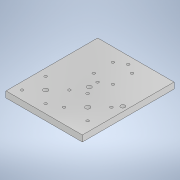
# Autodesk Inventor part: 14_XY_Plate
Saved by Autodesk Inventor 2022.2 (Build 262287010, 287A)
## iProperties
Created: 2022-04-30
Part Number: 14_XY_Plate
Material: Aluminium 6061
Document SubType Name: Modeling
Designer: MXBD
Density: 2.7 g/cm^3
Appearance: Aluminium - dunkel
Author: MXBD
Autodesk Inventor part; units mm, degrees
ref_plane "YZ Plane" through (0, 0, 0) normal (1, 0, 0) x (0, 1, 0)
ref_plane "XZ Plane" through (0, 0, 0) normal (0, 1, 0) x (-1, 0, 0)
ref_plane "XY Plane" through (0, 0, 0) normal (0, 0, 1) x (1, 0, 0)
sketch "Skizze1" plane through (0, 0, 0) normal (0, 1, 0) x (-1, 0, 0)
  line L0 (50, -60) -> (-50, -60)
  line L1 (-50, -60) -> (-50, 60)
  line L2 (-50, 60) -> (50, 60)
  line L3 (50, 60) -> (50, -60)
  line L4 (50, -60) -> (-50, 60) construction
  line L5 (-50, -60) -> (50, 60) construction
  point P0 (0, 0)
  dimension "d0" = 100
  dimension "d1" = 120
  constraints: 12 end point, 2 midpoint, 2 parallel, 1 horizontal, 1 perpendicular
  measures "d0" distance of L1.end L2.end
  measures "d1" distance of L0.end L1.end
extrude "Extrusion1" add sketch "Skizze1" along normal blind 8
sketch "Skizze2" plane through (0, 8, 0) normal (0, 1, 0) x (1, 0, 0)
  line L0 (-50, -60) -> (50, -60) projected
  line L1 (0, -60) -> (0, 152.9688)
  line L2 (50, 60) -> (-50, 60) projected
  point P0 (0, 0)
  point P1 (0, 10)
  point P2 (0, 50)
  dimension "d4" = 40
  dimension "d5" = 10
  constraints: 2 end point, 2 point on line, 1 midpoint, 1 vertical
  measures "d4" distance of point (0, 50) point (0, 10)
  measures "d5" distance from line of L2 point (0, 50)
hole "Rail_through_holes" at (0, 8, -10) at (0, 8, -50) direction (0, -1, 0) diameter 3.4 end through all clearance for "Inbusschraube ISO 4762" size "M3" standard "ISO"
sketch "Skizze3" plane through (0, 8, 0) normal (0, 1, 0) x (1, 0, 0)
  line L0 (-50, -60) -> (50, -60) projected
  line L1 (0, -60) -> (0, 60)
  line L2 (50, 60) -> (-50, 60) projected
  line L3 (12.5, 17.5) -> (-12.5, 17.5) construction
  line L4 (-12.5, 17.5) -> (-12.5, 42.5) construction
  line L5 (-12.5, 42.5) -> (12.5, 42.5) construction
  line L6 (12.5, 42.5) -> (12.5, 17.5) construction
  line L7 (12.5, 17.5) -> (-12.5, 42.5) construction
  line L8 (-12.5, 17.5) -> (12.5, 42.5) construction
  circle A0 centre (0, 50) radius 1.7 construction
  point P0 (0, 0)
  point P1 (0, 30)
  point P2 (0, 30)
  dimension "d13" = 25
  dimension "d14" = 25
  dimension "d15" = 20
  constraints: 14 end point, 5 midpoint, 4 coincident, 2 parallel, 1 horizontal, 1 perpendicular, 1 point on line
  measures "d13" distance of L4.end L5.end
  measures "d14" distance of L3.end L4.end
  measures "d15" distance of A0.centre point (0, 30)
hole "Slide_through_holes" at (-12.5, 8, -17.5) at (-12.5, 8, -42.5) at (12.5, 8, -42.5) at (12.5, 8, -17.5) direction (0, -1, 0) diameter 3.4 end through all clearance for "Inbusschraube ISO 4762" size "M3" standard "ISO"
sketch "Skizze4" plane through (0, 8, 0) normal (0, 1, 0) x (1, 0, 0)
  line L0 (-50, -60) -> (50, -60) projected
  line L1 (0, -60) -> (0, 74.7934)
  line L2 (-25, -60) -> (-25, 181.0187) construction
  line L3 (-9.5, -48.5) -> (-40.5, -48.5) construction
  line L4 (-40.5, -48.5) -> (-40.5, -17.5) construction
  line L5 (-40.5, -17.5) -> (-9.5, -17.5) construction
  line L6 (-9.5, -17.5) -> (-9.5, -48.5) construction
  line L7 (-9.5, -48.5) -> (-40.5, -17.5) construction
  line L8 (-40.5, -48.5) -> (-9.5, -17.5) construction
  line L9 (50, 60) -> (-50, 60) construction
  circle A0 centre (-25, -33) radius 3
  point P0 (0, 0)
  point P1 (-25, -33)
  dimension "d23" = 25
  dimension "d24" = 31
  dimension "d25" = 31
  dimension "d26" = 93
  dimension "d60" = 6
  constraints: 16 end point, 5 coincident, 4 midpoint, 2 parallel, 2 point on line, 2 vertical, 1 centre point, 1 horizontal, 1 perpendicular
  measures "d23" distance between parallel lines of L1 L2
  measures "d24" distance of L4.end L5.end
  measures "d25" distance of L3.end L4.end
  measures "d26" distance from line of L9 point (-25, -33)
  measures "d60" diameter of A0
hole "Nema_X_through_holes" at (-40.5, 8, 48.5) at (-40.5, 8, 17.5) at (-9.5, 8, 17.5) at (-9.5, 8, 48.5) direction (0, -1, 0) diameter 3.4 end through all clearance for "Inbusschraube ISO 4762" size "M3" standard "ISO"
extrude "Nema_X_Shaft" cut sketch "Skizze4" against normal through all
sketch "Skizze5" plane through (0, 8, 0) normal (0, 1, 0) x (1, 0, 0)
  line L0 (-50, -60) -> (50, -60) projected
  line L1 (0, -60) -> (0, 63.3778)
  line L2 (22, -60) -> (22, 63.3778) construction
  line L3 (37.5, -40.5) -> (6.5, -40.5) construction
  line L4 (6.5, -40.5) -> (6.5, -9.5) construction
  line L5 (6.5, -9.5) -> (37.5, -9.5) construction
  line L6 (37.5, -9.5) -> (37.5, -40.5) construction
  line L7 (37.5, -40.5) -> (6.5, -9.5) construction
  line L8 (6.5, -40.5) -> (37.5, -9.5) construction
  circle A0 centre (22, -25) radius 3
  line L9 (50, 60) -> (-50, 60) projected
  line L10 (0, 88.0534) -> (0, -84.6756) projected
  point P0 (0, 0)
  point P1 (4.5, 5)
  point P2 (39.5, 5)
  point P3 (22, -25)
  dimension "d34" = 22
  dimension "d35" = 31
  dimension "d36" = 31
  dimension "d47" = 85
  dimension "d48" = 35
  dimension "d49" = 30
  dimension "d59" = 6
  constraints: 16 end point, 6 coincident, 5 midpoint, 2 parallel, 2 point on line, 1 centre point, 1 collinear, 1 horizontal, 1 perpendicular, 1 symmetric about line, 1 other
  measures "d34" distance between parallel lines of L2 L1
  measures "d35" distance of L4.end L5.end
  measures "d36" distance of L3.end L4.end
  measures "d48" distance of point (39.5, 5) point (4.5, 5)
  measures "d49" vertical distance of point (4.5, 5) point (22, -25)
  measures "d59" diameter of A0
hole "Nema_Y_through_holes" at (6.5, 8, 40.5) at (6.5, 8, 9.5) at (37.5, 8, 9.5) at (37.5, 8, 40.5) direction (0, -1, 0) diameter 3.4 end through all clearance for "Inbusschraube ISO 4762" size "M3" standard "ISO"
extrude "Nema_Y_Shaft" cut sketch "Skizze5" against normal through all
sketch "Skizze6" plane through (0, 8, 0) normal (0, 1, 0) x (1, 0, 0)
  circle A0 centre (22, -25) radius 3 construction
  line L0 (22, -25) -> (22, 60.1123) construction
  line L1 (0, 84) -> (0, -84) construction
  point P0 (0, 0)
  point P1 (0, -1)
  point P2 (44, -1)
  dimension "d50" = 44
  dimension "d51" = 24
  constraints: 2 end point, 1 parallel, 1 symmetric about line, 1 vertical
  measures "d50" distance of point (0, -1) point (44, -1)
  measures "d51" vertical distance of L0.start point (0, -1)
hole "Y_Pulley_Shafts" at (0, 8, 1) at (44, 8, 1) direction (0, -1, 0) diameter 5.5 end through all clearance for "Inbusschraube ISO 4762" size "M5" standard "ISO"
